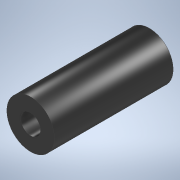
# Autodesk Inventor part: PlateSpacer
Saved by Autodesk Inventor 2020 (Build 240168000, 168)
## iProperties
Created: 2019-06-24
Part Number: PlateSpacer
Material: ABS Plastic
Document SubType Name: Modeling
Designer: Connor
Density: 1.06 g/cm^3
Appearance: Glossy - Black
Author: Connor
Autodesk Inventor part; units mm, degrees
ref_plane "YZ Plane" through (0, 0, 0) normal (1, 0, 0) x (0, 1, 0)
ref_plane "XZ Plane" through (0, 0, 0) normal (0, 1, 0) x (-1, 0, 0)
ref_plane "XY Plane" through (0, 0, 0) normal (0, 0, 1) x (1, 0, 0)
sketch "Sketch1" plane through (0, 0, 0) normal (0, 0, 1) x (1, 0, 0)
  circle A0 centre (0, 0) radius 2.667
  circle A1 centre (0, 0) radius 6.35
  dimension "d0" = 5.334
  dimension "d1" = 12.7
  constraints: 2 centre point, 2 coincident
  measures "d0" diameter of A0
  measures "d1" diameter of A1
extrude "Extrusion1" add sketch "Sketch1" along normal blind 31.75
body "Solid1"
